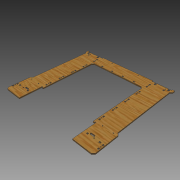
# Autodesk Inventor part: frame
Saved by Autodesk Inventor 2014 (Build 180170000, 170)
## iProperties
Created: 2013-12-06
Part Number: frame
Material: Plywood, Finish
Document SubType Name: Modeling
Designer: buben
Density: 0.552 g/cm^3
Appearance: Plywood - New
Author: buben
Subject: Laser Cutted
Autodesk Inventor part; units mm, degrees
ref_plane "YZ Plane" through (0, 0, 0) normal (1, 0, 0) x (0, 1, 0)
ref_plane "XZ Plane" through (0, 0, 0) normal (0, 1, 0) x (-1, 0, 0)
ref_plane "XY Plane" through (0, 0, 0) normal (0, 0, 1) x (1, 0, 0)
sketch "Sketch1" plane through (0, 0, 0) normal (0, 0, 1) x (1, 0, 0)
  line L0 (0, 528.5) -> (561, 528.5)
  line L1 (0, 10) -> (10, 0)
  line L2 (561, 10) -> (551, 0)
  line L3 (0, 511.5) -> (10, 501.5)
  line L4 (10, 501.5) -> (10, 140)
  line L5 (10, 140) -> (0, 130)
  line L6 (561, 511.5) -> (551, 501.5)
  line L7 (551, 501.5) -> (551, 140)
  line L8 (551, 140) -> (561, 130)
  line L9 (0, 10) -> (0, 130)
  line L10 (0, 511.5) -> (0, 528.5)
  line L11 (561, 528.5) -> (561, 511.5)
  line L12 (561, 130) -> (561, 10)
  line L13 (10, 0) -> (106, 0)
  line L14 (106, 0) -> (106, 123.5)
  line L15 (551, 0) -> (455, 0)
  line L16 (455, 0) -> (455, 123.5)
  line L17 (106, 123.5) -> (112.5, 123.5)
  line L18 (112.5, 123.5) -> (112.5, 119.5)
  line L19 (112.5, 119.5) -> (119, 119.5)
  line L20 (119, 119.5) -> (119, 438.5)
  line L21 (455, 123.5) -> (448.5, 123.5)
  line L22 (448.5, 123.5) -> (448.5, 119.5)
  line L23 (448.5, 119.5) -> (442, 119.5)
  line L24 (442, 119.5) -> (442, 438.5)
  line L25 (119, 438.5) -> (129, 448.5)
  line L26 (129, 448.5) -> (432, 448.5)
  line L27 (432, 448.5) -> (442, 438.5)
  point P0 (0, 0)
  point P1 (280.5, 448.5)
  point P2 (280.5, 528.5)
  dimension "d0" = 561
  dimension "d1" = 528.5
  dimension "d2" = 10
  dimension "d3" = 10
  dimension "d4" = 45
  dimension "d5" = 10
  dimension "d6" = 17
  dimension "d7" = 6.5
  dimension "d8" = 6.5
  dimension "d9" = 6.5
  dimension "d10" = 6.5
  dimension "d11" = 4
  dimension "d12" = 10
  dimension "d13" = 80
  dimension "d14" = 323
  dimension "d15" = 123.5
  dimension "d18" = 6.5
  constraints: 56 end point, 17 perpendicular, 12 parallel, 7 horizontal alignment, 3 vertical alignment, 2 collinear, 2 midpoint, 2 vertical
  measures "d0" distance of L0.start L0.end
  measures "d1" distance from line of L0 L1.end
  measures "d2" distance between parallel lines of L4 L10
  measures "d3" distance between parallel lines of L11 L7
  measures "d4" angle of L1 L13
  measures "d5" horizontal distance of L1.start L1.end
  measures "d6" distance of L3.start L0.start
  measures "d7" distance of L14.end L17.end
  measures "d8" distance of L16.end L21.end
  measures "d9" distance of L18.end L19.end
  measures "d10" distance of L22.end L23.end
  measures "d11" distance of L17.end L18.end
  measures "d12" horizontal distance of L20.end L25.end
  measures "d13" distance between parallel lines of L26 L0
  measures "d14" distance between parallel lines of L24 L20
  measures "d15" distance between parallel lines of L13 L17
  measures "d18" vertical distance of L14.end L5.end
extrude "Extrusion1" add sketch "Sketch1" along normal blind 6.5
sketch "Sketch15" plane through (0, 0, 6.5) normal (0, 0, 1) x (1, 0, 0)
  line L0 (561, 528.5) -> (0, 528.5) projected
  line L1 (0, 528.5) -> (0, 511.5) projected
  line L2 (561, 511.5) -> (561, 528.5) projected
  line L3 (12, 528.5) -> (118.5, 528.5)
  line L4 (118.5, 528.5) -> (118.5, 522)
  line L5 (118.5, 522) -> (12, 522)
  line L6 (12, 522) -> (12, 528.5)
  line L7 (442.5, 528.5) -> (549, 528.5)
  line L8 (549, 528.5) -> (549, 522)
  line L9 (549, 522) -> (442.5, 522)
  line L10 (442.5, 522) -> (442.5, 528.5)
  point P0 (0, 0)
  dimension "d138" = 6.5
  dimension "d139" = 12
  dimension "d141" = 12
  dimension "d145" = 106.5
  constraints: 16 end point, 4 parallel, 2 collinear, 2 horizontal, 2 perpendicular, 2 point on line
  measures "d138" distance of L3.end L4.end
  measures "d139" distance between parallel lines of L1 L6
  measures "d141" distance between parallel lines of L2 L8
  measures "d145" distance of L4.end L5.end
extrude "Extrusion15" cut sketch "Sketch15" against normal through all
sketch "Sketch16" plane through (0, 0, 6.5) normal (0, 0, 1) x (1, 0, 0)
  line L0 (442.5, 528.5) -> (118.5, 528.5) projected
  line L1 (119, 119.5) -> (119, 438.5) projected
  line L2 (129, 448.5) -> (432, 448.5) projected
  line L3 (280.5, 528.5) -> (280.5, 448.5) construction
  line L4 (106, 494) -> (112.5, 494)
  line L5 (112.5, 494) -> (112.5, 486)
  line L6 (112.5, 486) -> (106, 486)
  line L7 (106, 486) -> (106, 494)
  line L8 (106, 471) -> (112.5, 471)
  line L9 (112.5, 471) -> (112.5, 463)
  line L10 (112.5, 463) -> (106, 463)
  line L11 (106, 463) -> (106, 471)
  line L12 (106, 486) -> (112.5, 471) construction
  line L13 (106, 471) -> (112.5, 486) construction
  circle A0 centre (109.25, 478.5) radius 2.25
  line L14 (106, 414) -> (112.5, 414)
  line L15 (112.5, 414) -> (112.5, 406)
  line L16 (112.5, 406) -> (106, 406)
  line L17 (106, 406) -> (106, 414)
  line L18 (106, 391) -> (112.5, 391)
  line L19 (112.5, 391) -> (112.5, 383)
  line L20 (112.5, 383) -> (106, 383)
  line L21 (106, 383) -> (106, 391)
  line L22 (106, 406) -> (112.5, 391) construction
  line L23 (106, 391) -> (112.5, 406) construction
  circle A1 centre (109.25, 398.5) radius 2.25
  line L24 (106, 334) -> (112.5, 334)
  line L25 (112.5, 334) -> (112.5, 326)
  line L26 (112.5, 326) -> (106, 326)
  line L27 (106, 326) -> (106, 334)
  line L28 (106, 311) -> (112.5, 311)
  line L29 (112.5, 311) -> (112.5, 303)
  line L30 (112.5, 303) -> (106, 303)
  line L31 (106, 303) -> (106, 311)
  line L32 (106, 326) -> (112.5, 311) construction
  line L33 (106, 311) -> (112.5, 326) construction
  circle A2 centre (109.25, 318.5) radius 2.25
  line L34 (106, 254) -> (112.5, 254)
  line L35 (112.5, 254) -> (112.5, 246)
  line L36 (112.5, 246) -> (106, 246)
  line L37 (106, 246) -> (106, 254)
  line L38 (106, 231) -> (112.5, 231)
  line L39 (112.5, 231) -> (112.5, 223)
  line L40 (112.5, 223) -> (106, 223)
  line L41 (106, 223) -> (106, 231)
  line L42 (106, 246) -> (112.5, 231) construction
  line L43 (106, 231) -> (112.5, 246) construction
  circle A3 centre (109.25, 238.5) radius 2.25
  line L44 (106, 174) -> (112.5, 174)
  line L45 (112.5, 174) -> (112.5, 166)
  line L46 (112.5, 166) -> (106, 166)
  line L47 (106, 166) -> (106, 174)
  line L48 (106, 151) -> (112.5, 151)
  line L49 (112.5, 151) -> (112.5, 143)
  line L50 (112.5, 143) -> (106, 143)
  line L51 (106, 143) -> (106, 151)
  line L52 (106, 166) -> (112.5, 151) construction
  line L53 (106, 151) -> (112.5, 166) construction
  circle A4 centre (109.25, 158.5) radius 2.25
  line L54 (455, 494) -> (448.5, 494)
  line L55 (448.5, 494) -> (448.5, 486)
  line L56 (448.5, 486) -> (455, 486)
  line L57 (455, 486) -> (455, 494)
  line L58 (455, 471) -> (448.5, 471)
  line L59 (448.5, 471) -> (448.5, 463)
  line L60 (448.5, 463) -> (455, 463)
  line L61 (455, 463) -> (455, 471)
  line L62 (455, 486) -> (448.5, 471) construction
  line L63 (455, 471) -> (448.5, 486) construction
  circle A5 centre (451.75, 478.5) radius 2.25
  line L64 (448.5, 383) -> (455, 383)
  line L65 (455, 383) -> (455, 391)
  line L66 (455, 391) -> (448.5, 391)
  line L67 (448.5, 391) -> (448.5, 383)
  circle A6 centre (451.75, 398.5) radius 2.25
  line L68 (448.5, 406) -> (455, 406)
  line L69 (455, 406) -> (448.5, 391) construction
  line L70 (455, 391) -> (448.5, 406) construction
  line L71 (455, 406) -> (455, 414)
  line L72 (455, 414) -> (448.5, 414)
  line L73 (448.5, 414) -> (448.5, 406)
  line L74 (448.5, 303) -> (455, 303)
  line L75 (455, 303) -> (455, 311)
  line L76 (455, 311) -> (448.5, 311)
  line L77 (448.5, 311) -> (448.5, 303)
  circle A7 centre (451.75, 318.5) radius 2.25
  line L78 (448.5, 326) -> (455, 326)
  line L79 (455, 326) -> (448.5, 311) construction
  line L80 (455, 311) -> (448.5, 326) construction
  line L81 (455, 326) -> (455, 334)
  line L82 (455, 334) -> (448.5, 334)
  line L83 (448.5, 334) -> (448.5, 326)
  line L84 (448.5, 223) -> (455, 223)
  line L85 (455, 223) -> (455, 231)
  line L86 (455, 231) -> (448.5, 231)
  line L87 (448.5, 231) -> (448.5, 223)
  circle A8 centre (451.75, 238.5) radius 2.25
  line L88 (448.5, 246) -> (455, 246)
  line L89 (455, 246) -> (448.5, 231) construction
  line L90 (455, 231) -> (448.5, 246) construction
  line L91 (455, 246) -> (455, 254)
  line L92 (455, 254) -> (448.5, 254)
  line L93 (448.5, 254) -> (448.5, 246)
  line L94 (448.5, 143) -> (455, 143)
  line L95 (455, 143) -> (455, 151)
  line L96 (455, 151) -> (448.5, 151)
  line L97 (448.5, 151) -> (448.5, 143)
  circle A9 centre (451.75, 158.5) radius 2.25
  line L98 (448.5, 166) -> (455, 166)
  line L99 (455, 166) -> (448.5, 151) construction
  line L100 (455, 151) -> (448.5, 166) construction
  line L101 (455, 166) -> (455, 174)
  line L102 (455, 174) -> (448.5, 174)
  line L103 (448.5, 174) -> (448.5, 166)
  line L104 (112.5, 123.5) -> (112.5, 119.5) projected
  point P0 (0, 0)
  dimension "d146" = 6.5
  dimension "d147" = 8
  dimension "d148" = 15
  dimension "d149" = 4.5
  dimension "d151" = 50
  dimension "d154" = 80
  constraints: 202 end point, 45 symmetric about line, 10 centre point, 4 collinear, 4 parallel, 3 midpoint, 2 horizontal, 2 perpendicular, 1 vertical, 85 other
  measures "d146" distance of L4.start L4.end
  measures "d147" distance of L6.end L4.start
  measures "d148" distance between parallel lines of L8 L6
  measures "d149" diameter of A0
  measures "d151" distance from line of L0 A0.centre
  measures "d154" distance of L10.end L20.end
extrude "Extrusion16" cut sketch "Sketch16" against normal through all
sketch "Sketch17" plane through (0, 0, 6.5) normal (0, 0, 1) x (1, 0, 0)
  line L0 (129, 448.5) -> (432, 448.5) projected
  line L1 (173.3, 461) -> (181.3, 461)
  line L2 (181.3, 461) -> (181.3, 454.5)
  line L3 (181.3, 454.5) -> (173.3, 454.5)
  line L4 (173.3, 454.5) -> (173.3, 461)
  line L5 (242.1, 461) -> (250.1, 461)
  line L6 (250.1, 461) -> (250.1, 454.5)
  line L7 (250.1, 454.5) -> (242.1, 454.5)
  line L8 (242.1, 454.5) -> (242.1, 461)
  line L9 (310.9, 461) -> (318.9, 461)
  line L10 (318.9, 461) -> (318.9, 454.5)
  line L11 (318.9, 454.5) -> (310.9, 454.5)
  line L12 (310.9, 454.5) -> (310.9, 461)
  line L13 (379.7, 461) -> (387.7, 461)
  line L14 (387.7, 461) -> (387.7, 454.5)
  line L15 (387.7, 454.5) -> (379.7, 454.5)
  line L16 (379.7, 454.5) -> (379.7, 461)
  line L17 (173.3, 457.75) -> (112.5, 457.75) construction
  line L18 (181.3, 457.75) -> (242.1, 457.75) construction
  line L19 (250.1, 457.75) -> (310.9, 457.75) construction
  line L20 (318.9, 457.75) -> (379.7, 457.75) construction
  line L21 (387.7, 457.75) -> (448.5, 457.75) construction
  point P0 (112.5, 463)
  point P1 (448.5, 463)
  point P2 (0, 0)
  dimension "d161" = 8
  dimension "d162" = 6.5
  dimension "d163" = 6
  constraints: 42 end point, 13 collinear, 9 equal length, 8 midpoint, 5 perpendicular, 4 horizontal, 2 vertical alignment
  measures "d161" distance of L1.start L1.end
  measures "d162" distance of L3.end L1.start
  measures "d163" distance between parallel lines of L0 L3
extrude "Extrusion17" cut sketch "Sketch17" against normal through all
sketch "Sketch18" plane through (0, 0, 6.5) normal (0, 0, 1) x (1, 0, 0)
  line L0 (442.5, 528.5) -> (118.5, 528.5) projected
  circle A0 centre (195.75, 515.5) radius 2.25
  circle A1 centre (365.25, 515.5) radius 2.25
  line L1 (448.5, 486) -> (448.5, 494) projected
  line L2 (112.5, 494) -> (112.5, 486) projected
  point P0 (0, 0)
  dimension "d166" = 13
  dimension "d167" = 4.5
  dimension "d197" = 83.25
  dimension "d198" = 83.25
  constraints: 2 centre point, 1 equal radius, 1 horizontal alignment
  measures "d166" distance from line of L0 A0.centre
  measures "d167" diameter of A0
  measures "d197" distance from line of L2 A0.centre
  measures "d198" distance from line of L1 A1.centre
extrude "Extrusion18" cut sketch "Sketch18" against normal through all
sketch "Sketch19" plane through (0, 0, 6.5) normal (0, 0, 1) x (1, 0, 0)
  line L0 (442.5, 528.5) -> (118.5, 528.5) projected
  line L1 (0, 130) -> (0, 10) projected
  line L2 (106, 123.5) -> (112.5, 123.5) projected
  line L3 (129, 448.5) -> (432, 448.5) projected
  line L4 (3, 59.5) -> (9.5, 59.5)
  line L5 (9.5, 59.5) -> (9.5, 51.5)
  line L6 (9.5, 51.5) -> (3, 51.5)
  line L7 (3, 51.5) -> (3, 59.5)
  line L8 (3, 36.5) -> (9.5, 36.5)
  line L9 (9.5, 36.5) -> (9.5, 28.5)
  line L10 (9.5, 28.5) -> (3, 28.5)
  line L11 (3, 28.5) -> (3, 36.5)
  circle A0 centre (6.25, 44) radius 2.25
  line L12 (280.5, 528.5) -> (280.5, 448.5) construction
  line L13 (558, 59.5) -> (551.5, 59.5)
  line L14 (551.5, 59.5) -> (551.5, 51.5)
  line L15 (551.5, 51.5) -> (558, 51.5)
  line L16 (558, 51.5) -> (558, 59.5)
  line L17 (558, 36.5) -> (551.5, 36.5)
  line L18 (551.5, 36.5) -> (551.5, 28.5)
  line L19 (551.5, 28.5) -> (558, 28.5)
  line L20 (558, 28.5) -> (558, 36.5)
  circle A1 centre (554.75, 44) radius 2.25
  point P0 (0, 0)
  point P1 (6.25, 51.5)
  point P2 (554.75, 51.5)
  dimension "d172" = 6.5
  dimension "d173" = 8
  dimension "d174" = 15
  dimension "d175" = 7.5
  dimension "d176" = 3
  dimension "d178" = 4.5
  dimension "d181" = 79.5
  constraints: 34 end point, 10 symmetric about line, 4 parallel, 3 collinear, 3 midpoint, 2 centre point, 2 horizontal, 2 perpendicular, 1 vertical alignment, 1 other
  measures "d172" distance of L9.end L10.end
  measures "d173" distance of L10.end L8.start
  measures "d174" distance between parallel lines of L8 L6
  measures "d175" distance from line of A0.centre L6
  measures "d176" distance between parallel lines of L1 L7
  measures "d178" diameter of A0
  measures "d181" distance from line of A0.centre L2
extrude "Extrusion19" cut sketch "Sketch19" against normal through all
sketch "Sketch20" plane through (0, 0, 6.5) normal (0, 0, 1) x (1, 0, 0)
  line L0 (442.5, 528.5) -> (118.5, 528.5) projected
  line L1 (0, 130) -> (0, 10) projected
  line L2 (10, 0) -> (106, 0) projected
  line L3 (106, 0) -> (106, 123.5) projected
  line L4 (129, 448.5) -> (432, 448.5) projected
  line L5 (20, 61) -> (28, 61)
  line L6 (28, 61) -> (28, 54.5)
  line L7 (28, 54.5) -> (20, 54.5)
  line L8 (20, 54.5) -> (20, 61)
  line L9 (83, 61) -> (91, 61)
  line L10 (91, 61) -> (91, 54.5)
  line L11 (91, 54.5) -> (83, 54.5)
  line L12 (83, 54.5) -> (83, 61)
  circle A0 centre (53, 57.75) radius 2.25
  line L13 (280.5, 528.5) -> (280.5, 448.5) construction
  line L14 (541, 61) -> (533, 61)
  line L15 (533, 61) -> (533, 54.5)
  line L16 (533, 54.5) -> (541, 54.5)
  line L17 (541, 54.5) -> (541, 61)
  line L18 (478, 61) -> (470, 61)
  line L19 (470, 61) -> (470, 54.5)
  line L20 (470, 54.5) -> (478, 54.5)
  line L21 (478, 54.5) -> (478, 61)
  circle A1 centre (508, 57.75) radius 2.25
  point P0 (0, 0)
  point P1 (28, 57.75)
  point P2 (533, 57.75)
  dimension "d182" = 6.5
  dimension "d183" = 8
  dimension "d184" = 4.5
  dimension "d185" = 20
  dimension "d186" = 15
  dimension "d187" = 53
  dimension "d188" = 54.5
  constraints: 34 end point, 10 symmetric about line, 4 parallel, 3 collinear, 3 midpoint, 2 centre point, 2 horizontal, 2 perpendicular, 1 horizontal alignment, 1 other
  measures "d182" distance of L7.end L5.start
  measures "d183" distance of L5.start L5.end
  measures "d184" diameter of A0
  measures "d185" distance between parallel lines of L1 L8
  measures "d186" distance between parallel lines of L3 L10
  measures "d187" distance from line of L3 A0.centre
  measures "d188" distance between parallel lines of L2 L11
extrude "Extrusion20" cut sketch "Sketch20" against normal through all
sketch "Sketch21" plane through (0, 0, 6.5) normal (0, 0, 1) x (1, 0, 0)
  line L0 (442.5, 528.5) -> (118.5, 528.5) projected
  line L1 (0, 130) -> (0, 10) projected
  line L2 (129, 448.5) -> (432, 448.5) projected
  circle A0 centre (20, 126.75) radius 2.25
  circle A1 centre (75, 126.75) radius 2.25
  line L3 (280.5, 528.5) -> (280.5, 448.5) construction
  circle A2 centre (541, 126.75) radius 2.25
  circle A3 centre (486, 126.75) radius 2.25
  point P0 (0, 0)
  dimension "d191" = 4.5
  dimension "d192" = 55
  dimension "d193" = 20
  dimension "d194" = 3.25
  constraints: 4 centre point, 2 end point, 2 midpoint, 2 symmetric about line, 1 equal radius, 1 horizontal alignment, 2 other
  measures "d191" diameter of A0
  measures "d192" distance of A1.centre A0.centre
  measures "d193" distance from line of L1 A0.centre
  measures "d194" vertical distance of L1.start A0.centre
extrude "Extrusion21" cut sketch "Sketch21" against normal through all
chamfer "Chamfer1" distance 3 angle 45 1 edges at (119, 119.5, 3.25)
sketch "Sketch22" plane through (0, 0, 6.5) normal (0, 0, 1) x (1, 0, 0)
  line L0 (129, 448.5) -> (432, 448.5) projected
  line L1 (442.5, 528.5) -> (118.5, 528.5) projected
  line L2 (20, 61) -> (28, 61) projected
  line L3 (83, 54.5) -> (83, 61) projected
  line L4 (280.5, 528.5) -> (280.5, 448.5) construction
  line L5 (61.5, 66) -> (76.5, 66) construction
  line L6 (61.5, 62) -> (76.5, 62)
  line L7 (76.5, 70) -> (61.5, 70)
  arc A0 (61.5, 70) -> (61.5, 62) centre (61.5, 66) ccw
  arc A1 (76.5, 62) -> (76.5, 70) centre (76.5, 66) ccw
  line L8 (499.5, 66) -> (484.5, 66) construction
  line L9 (499.5, 62) -> (484.5, 62)
  line L10 (484.5, 70) -> (499.5, 70)
  arc A2 (499.5, 62) -> (499.5, 70) centre (499.5, 66) ccw
  arc A3 (484.5, 70) -> (484.5, 62) centre (484.5, 66) ccw
  point P0 (0, 0)
  point P1 (69, 66)
  point P2 (492, 66)
  dimension "d202" = 8
  dimension "d203" = 15
  dimension "d206" = 1
  dimension "d207" = 14
  constraints: 18 end point, 8 point on circle, 7 symmetric about line, 4 centre point, 4 tangent, 3 midpoint, 1 parallel, 1 perpendicular, 2 other
  measures "d202" distance between parallel lines of L7 L6
  measures "d203" distance of L5.start L5.end
  measures "d206" distance between parallel lines of L2 L6
  measures "d207" distance from line of L3 point (69, 66)
extrude "Extrusion22" cut sketch "Sketch22" against normal through all
sketch "Sketch23" plane through (0, 0, 6.5) normal (0, 0, 1) x (1, 0, 0)
  line L0 (129, 448.5) -> (432, 448.5) projected
  line L1 (442.5, 528.5) -> (118.5, 528.5) projected
  line L2 (118.5, 522) -> (12, 522) projected
  line L3 (0, 528.5) -> (0, 511.5) projected
  line L4 (280.5, 528.5) -> (280.5, 448.5) construction
  line L5 (19.967, 522) -> (24.467, 522)
  line L6 (24.467, 505.7) -> (19.967, 505.7)
  line L7 (26.967, 517) -> (26.967, 509.7)
  line L8 (17.467, 509.7) -> (17.467, 517)
  line L9 (17.467, 517) -> (19.967, 517)
  line L10 (24.467, 517) -> (26.967, 517)
  line L11 (19.967, 505.7) -> (19.967, 509.7)
  line L12 (19.967, 517) -> (19.967, 522)
  line L13 (26.967, 509.7) -> (24.467, 509.7)
  line L14 (19.967, 509.7) -> (17.467, 509.7)
  line L15 (24.467, 522) -> (24.467, 517)
  line L16 (24.467, 509.7) -> (24.467, 505.7)
  line L17 (541.033, 522) -> (536.533, 522)
  line L18 (536.533, 505.7) -> (541.033, 505.7)
  line L19 (534.033, 517) -> (534.033, 509.7)
  line L20 (543.533, 509.7) -> (543.533, 517)
  line L21 (543.533, 517) -> (541.033, 517)
  line L22 (536.533, 517) -> (534.033, 517)
  line L23 (541.033, 505.7) -> (541.033, 509.7)
  line L24 (541.033, 517) -> (541.033, 522)
  line L25 (534.033, 509.7) -> (536.533, 509.7)
  line L26 (541.033, 509.7) -> (543.533, 509.7)
  line L27 (536.533, 522) -> (536.533, 517)
  line L28 (536.533, 509.7) -> (536.533, 505.7)
  point P0 (0, 0)
  point P1 (22.217, 505.7)
  point P2 (538.783, 505.7)
  dimension "d210" = 4.5
  dimension "d211" = 5
  dimension "d212" = 4
  dimension "d213" = 7.3
  dimension "d214" = 2.5
  dimension "d215" = 22.217
  constraints: 50 end point, 13 symmetric about line, 10 parallel, 6 collinear, 4 perpendicular, 3 horizontal, 3 midpoint
  measures "d210" distance of L6.start L6.end
  measures "d211" distance of L5.end L10.start
  measures "d212" distance of L13.end L6.start
  measures "d213" distance of L7.start L7.end
  measures "d214" distance of L11.end L8.start
  measures "d215" distance from line of point (22.217, 505.7) L3
extrude "Extrusion23" cut sketch "Sketch23" against normal through all
sketch "Sketch24" plane through (0, 0, 6.5) normal (0, 0, 1) x (1, 0, 0)
  line L0 (106, 463) -> (106, 471) projected
  line L1 (106, 471) -> (112.5, 471) projected
  circle A0 centre (109.25, 478.5) radius 2.25 projected
  line L2 (12, 528.5) -> (0, 528.5) projected
  line L3 (0, 528.5) -> (0, 511.5) projected
  line L4 (129, 448.5) -> (432, 448.5) projected
  line L5 (442.5, 528.5) -> (118.5, 528.5) projected
  circle A1 centre (38.078, 510.5) radius 2.25
  line L6 (34.828, 500.5) -> (41.328, 500.5)
  line L7 (41.328, 500.5) -> (41.328, 492.5)
  line L8 (41.328, 492.5) -> (34.828, 492.5)
  line L9 (34.828, 492.5) -> (34.828, 500.5)
  line L10 (280.5, 528.5) -> (280.5, 448.5) construction
  circle A2 centre (522.922, 510.5) radius 2.25
  line L11 (526.172, 500.5) -> (519.672, 500.5)
  line L12 (519.672, 500.5) -> (519.672, 492.5)
  line L13 (519.672, 492.5) -> (526.172, 492.5)
  line L14 (526.172, 492.5) -> (526.172, 500.5)
  point P0 (0, 0)
  point P1 (38.078, 500.5)
  point P2 (522.922, 500.5)
  dimension "d218" = 10
  dimension "d219" = 18
  dimension "d220" = 38.078
  constraints: 18 end point, 6 symmetric about line, 4 parallel, 3 midpoint, 2 centre point, 1 equal radius, 1 horizontal, 1 perpendicular, 1 vertical alignment, 1 other
  measures "d218" distance from line of L6 A1.centre
  measures "d219" distance from line of A1.centre L2
  measures "d220" distance from line of L3 A1.centre
extrude "Extrusion24" cut sketch "Sketch24" against normal through all contours A1 | L6 L7 L8 L9 | A2 | L14 L13 L12 L11
sketch "Sketch25" plane through (0, 0, 6.5) normal (0, 0, 1) x (1, 0, 0)
  line L0 (129, 448.5) -> (432, 448.5) projected
  line L1 (442.5, 528.5) -> (118.5, 528.5) projected
  line L2 (118.5, 528.5) -> (118.5, 522) projected
  line L3 (118.5, 522) -> (24.467, 522) projected
  line L4 (91.25, 522) -> (95.75, 522)
  line L5 (95.75, 505.7) -> (91.25, 505.7)
  line L6 (98.25, 517) -> (98.25, 509.7)
  line L7 (88.75, 509.7) -> (88.75, 517)
  line L8 (91.25, 505.7) -> (91.25, 509.7)
  line L9 (91.25, 517) -> (91.25, 522)
  line L10 (95.75, 522) -> (95.75, 517)
  line L11 (95.75, 509.7) -> (95.75, 505.7)
  line L12 (88.75, 517) -> (91.25, 517)
  line L13 (95.75, 517) -> (98.25, 517)
  line L14 (98.25, 509.7) -> (95.75, 509.7)
  line L15 (91.25, 509.7) -> (88.75, 509.7)
  line L16 (280.5, 528.5) -> (280.5, 448.5) construction
  line L17 (469.75, 522) -> (465.25, 522)
  line L18 (465.25, 505.7) -> (469.75, 505.7)
  line L19 (462.75, 517) -> (462.75, 509.7)
  line L20 (472.25, 509.7) -> (472.25, 517)
  line L21 (469.75, 505.7) -> (469.75, 509.7)
  line L22 (469.75, 517) -> (469.75, 522)
  line L23 (465.25, 522) -> (465.25, 517)
  line L24 (465.25, 509.7) -> (465.25, 505.7)
  line L25 (472.25, 517) -> (469.75, 517)
  line L26 (465.25, 517) -> (462.75, 517)
  line L27 (462.75, 509.7) -> (465.25, 509.7)
  line L28 (469.75, 509.7) -> (472.25, 509.7)
  point P0 (0, 0)
  point P1 (93.5, 505.7)
  point P2 (467.5, 505.7)
  dimension "d223" = 4.5
  dimension "d224" = 7.3
  dimension "d225" = 5
  dimension "d226" = 4
  dimension "d227" = 2.5
  dimension "d228" = 25
  constraints: 50 end point, 13 symmetric about line, 10 parallel, 6 collinear, 4 perpendicular, 3 horizontal, 3 midpoint
  measures "d223" distance of L5.start L5.end
  measures "d224" distance of L7.start L7.end
  measures "d225" distance of L9.start L4.start
  measures "d226" distance of L5.end L8.end
  measures "d227" distance of L8.end L7.start
  measures "d228" distance from line of L2 point (93.5, 505.7)
extrude "Extrusion25" cut sketch "Sketch25" against normal through all
equation "\"d3\" = d2"
equation "\"d8\" = d7"
equation "\"d9\" = d7"
equation "\"d10\" = d8"
body "Solid1"
